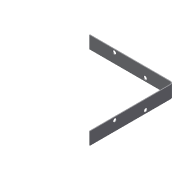
# Autodesk Inventor part: 80mmCornerBracket
Saved by Autodesk Inventor 2017 (Build 210142000, 142)
## iProperties
Created: 2015-04-22
Part Number: 80mmCornerBracket
Material: Generic
Document SubType Name: Modeling
Designer: krosie
Density: 1 g/cm^3
Appearance: Default
Author: krosie
Autodesk Inventor part; units mm, degrees
ref_plane "YZ Plane" through (0, 0, 0) normal (1, 0, 0) x (0, 1, 0)
ref_plane "XZ Plane" through (0, 0, 0) normal (0, 1, 0) x (-1, 0, 0)
ref_plane "XY Plane" through (0, 0, 0) normal (0, 0, 1) x (1, 0, 0)
sketch "Sketch1" plane through (0, 0, 0) normal (0, 0, 1) x (1, 0, 0)
  line L0 (0, 0) -> (97, 0)
  line L1 (100, -3) -> (100, -100)
  arc A0 (100, -3) -> (97, 0) centre (97, -3) ccw
  point P0 (100, 0)
  dimension "d0" = 100
  dimension "d1" = 100
  dimension "d7" = 3
  constraints: 4 end point, 2 point on circle, 2 point on line, 2 tangent, 1 centre point, 1 horizontal, 1 perpendicular
  measures "d0" distance of L0.start point (100, 0)
  measures "d1" distance of point (100, 0) L1.end
  measures "d7" radius of A0
sketch "Sketch2" plane through (0, 0, 0) normal (1, 0, 0) x (0, 1, 0)
  line L0 (0, 0) -> (0, -15)
  line L1 (0, -15) -> (1, -15)
  line L2 (1, -15) -> (1, 0)
  line L3 (1, 0) -> (0, 0)
  dimension "d2" = 15
  dimension "d3" = 1
  dimension "d4" = 15
  constraints: 8 end point, 2 perpendicular, 1 vertical
  measures "d2" distance of L0.start L0.end
  measures "d3" distance of L0.end L1.end
  measures "d4" distance of L1.end L2.end
sweep "Sweep1" add profiles "Sketch2" path "Sketch1"
hole "Hole1" at (30, 1, -3.5) direction (0, -1, 0) diameter 4 end through all
hole "Hole2" at (67, 1, -11.5) direction (0, -1, 0) diameter 4 end through all
hole "Hole3" at (101, -33, -11.5) direction (-1, 0, 0) diameter 4 end through all
hole "Hole4" at (101, -70, -3.5) direction (-1, 0, 0) diameter 4 end through all
chamfer "Chamfer1" distance 0.25 angle 45 4 edges at (30, 0, -5.5) (67, 0, -13.5) (100, -33, -9.5) (100, -70, -1.5)
body "Solid1"
